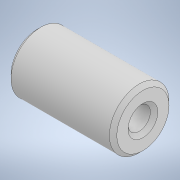
# Autodesk Inventor part: Rear Fan Spacer
Saved by Autodesk Inventor 2020 (Build 240168000, 168)
## iProperties
Created: 2019-12-21
Part Number: Rear Fan Spacer
Material: Generic
Document SubType Name: Modeling
Designer: pepd9
Density: 1 g/cm^3
Appearance: Default
Mass: 0.59077 g
Surface Area: 5.63474 cm^2
Volume: 0.59077 cm^3
Author: pepd9
Autodesk Inventor part; units mm, degrees
ref_plane "YZ Plane" through (0, 0, 0) normal (1, 0, 0) x (0, 1, 0)
ref_plane "XZ Plane" through (0, 0, 0) normal (0, 1, 0) x (-1, 0, 0)
ref_plane "XY Plane" through (0, 0, 0) normal (0, 0, 1) x (1, 0, 0)
sketch "Sketch1" plane through (0, 0, 0) normal (1, 0, 0) x (0, 1, 0)
  circle A0 centre (0, 0) radius 4
  dimension "d0" = 8
  constraints: 1 centre point, 1 coincident
  measures "d0" diameter of A0
extrude "Extrusion1" add sketch "Sketch1" along normal blind 14.2
sketch "Sketch2" plane through (14.2, 0, 0) normal (1, 0, 0) x (0, 0, -1)
  circle A0 centre (0, 0) radius 4 projected
hole "Hole1" at (14.2, 0, 0) direction (-1, 0, 0) diameter 3 end through all clearance for "Socket Head Cap Screw" size "M3" standard "Ansi Metric M Profile"
chamfer "Chamfer1" distance 0.5 angle 45 4 edges at (0, -4, 0) (0, 0, 1.5) (14.2, 0, 1.5) (14.2, -4, 0)
body "Solid1"
